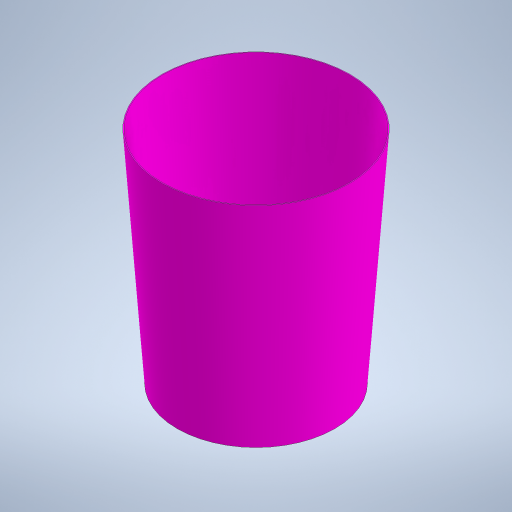
# Autodesk Inventor part: C
Saved by Autodesk Inventor 2024 (Build 280153000, 153)
## iProperties
Created: 2024-05-08
Part Number: C
Material: Generic
Document SubType Name: Modeling
Designer: VIJAY
Density: 1 g/cm^3
Appearance: Default
Author: VIJAY
Autodesk Inventor part; units mm, degrees
ref_plane "YZ Plane" through (0, 0, 0) normal (1, 0, 0) x (0, 1, 0)
ref_plane "XZ Plane" through (0, 0, 0) normal (0, 1, 0) x (-1, 0, 0)
ref_plane "XY Plane" through (0, 0, 0) normal (0, 0, 1) x (1, 0, 0)
sketch "Sketch1" plane through (0, 0, 0) normal (0, 1, 0) x (-1, 0, 0)
  circle A0 centre (0, 0) radius 35.76
  dimension "d0" = 71.52
  constraints: 1 centre point, 1 coincident
  measures "d0" diameter of A0
extrude "Extrusion1" add sketch "Sketch1" along normal blind 100 draft 4
shell "Shell1" thickness 0.38 removed faces 2 at (12.263, 0, 4.9679) at (-12.4499, 100, -11.2099)
body "Solid1"
